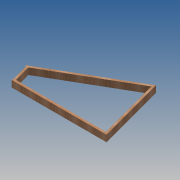
# Autodesk Inventor part: panelAflat
Saved by Autodesk Inventor 2014 SP1 (Build 180222100, 222)
## iProperties
Created: 2015-02-12
Part Number: panelAflat
Material: Wood (Birch)
Document SubType Name: Modeling
Designer: Dave
Density: 0.55 g/cm^3
Appearance: Birch - Natural Polished
Mass: 11299.2 g
Surface Area: 14418.2 cm^2
Volume: 20544 cm^3
Author: Dave
Autodesk Inventor part; units mm, degrees
ref_plane "YZ Plane" through (0, 0, 0) normal (1, 0, 0) x (0, 1, 0)
ref_plane "XZ Plane" through (0, 0, 0) normal (0, 1, 0) x (-1, 0, 0)
ref_plane "XY Plane" through (0, 0, 0) normal (0, 0, 1) x (1, 0, 0)
sketch "Sketch1" plane through (0, 0, 0) normal (0, 1, 0) x (-1, 0, 0)
  line L0 (0, 0) -> (-3000, 0) construction
  line L1 (0, 0) -> (-2598.0762, -1500) construction
  line L2 (0, 0) -> (3000, 0) construction
  arc A0 (-497.4937, 50) -> (-402.0602, -297.2332) centre (0, 0) ccw
  line L3 (-497.4937, 50) -> (-2157.4937, 50)
  line L4 (-2157.4937, 50) -> (-1841.7345, -1128.4295)
  line L5 (-2157.4937, 50) -> (-937.4937, 50) construction
  line L6 (-1841.7345, -1128.4295) -> (1158.2655, -1128.4295) construction
  line L7 (-1841.7345, -1128.4295) -> (-402.0602, -297.2332)
  arc A1 (-537.8662, 12) -> (-456.459, -284.7617) centre (0, 0) ccw
  line L8 (-2107.9712, 12) -> (-537.8662, 12)
  line L9 (-456.459, -284.7617) -> (-1817.8467, -1070.7593)
  line L10 (-2107.9712, 12) -> (-1817.8467, -1070.7593)
  dimension "d1" = 3000
  dimension "d2" = 150
  dimension "d3" = 1000
  dimension "d11" = 50
  dimension "d12" = 1660
  dimension "d13" = 1220
  dimension "d14" = 75
  constraints: 22 end point, 4 horizontal, 4 point on circle, 3 parallel, 2 centre point, 2 equal length, 1 coincident
  measures "d1" distance of L0.start L1.end
  measures "d2" angle of L1 L2
  measures "d3" diameter of A0
  measures "d11" distance between parallel lines of L3 L0
  measures "d12" distance of L3.start L3.end
  measures "d13" distance of L3.end L4.end
  measures "d14" angle of L4 L5
extrude "Extrusion2" add sketch "Sketch1" along normal blind 114
sketch "Sketch2" plane through (0, 114, 0) normal (0, 1, 0) x (1, 0, 0)
  line L0 (497.4937, -50) -> (2157.4937, -50) projected
  line L1 (1841.7345, 1128.4295) -> (402.0602, 297.2332) projected
  arc A0 (497.4937, -50) -> (402.0602, 297.2332) centre (0, 0) ccw projected
  line L2 (456.459, 284.7617) -> (537.8662, -12)
  line L3 (456.459, 284.7617) -> (423.5293, 265.7497)
  line L4 (537.8662, -12) -> (499.856, -12)
  line L5 (423.5293, 265.7497) -> (499.856, -12)
  constraints: 8 end point, 2 parallel, 2 point on circle
extrude "Extrusion3" add sketch "Sketch2" against normal blind 114 contours L5 A0
sketch "Sketch3" plane through (0, 114, 0) normal (0, 1, 0) x (1, 0, 0)
  arc A0 (537.8662, -12) -> (456.459, 284.7617) centre (0, 0) ccw projected
  line L0 (456.459, 284.7617) -> (537.8662, -12)
  constraints: 2 end point
extrude "Extrusion4" cut sketch "Sketch3" against normal blind 3500
sketch "Sketch4" plane through (0, 114, 0) normal (0, 1, 0) x (1, 0, 0)
  line L0 (537.8662, -12) -> (456.459, 284.7617) projected
  line L1 (2107.9712, -12) -> (537.8662, -12) projected
  line L2 (1841.7345, 1128.4295) -> (402.0602, 297.2332) projected
  line L3 (423.5293, 265.7497) -> (499.856, -12) projected
  line L4 (456.459, 284.7617) -> (423.5293, 265.7497)
  line L5 (499.856, -12) -> (537.8662, -12)
  constraints: 4 end point, 1 collinear, 1 parallel
extrude "Extrusion5" cut sketch "Sketch4" against normal blind 1
sketch "Sketch5" plane through (0, 114, 0) normal (0, 1, 0) x (1, 0, 0)
  line L0 (1817.8467, 1070.7593) -> (2107.9712, -12) projected
  line L1 (497.4937, -50) -> (2157.4937, -50) projected
  line L2 (2157.4937, -50) -> (1841.7345, 1128.4295) projected
  line L3 (1841.7345, 1128.4295) -> (402.0602, 297.2332) projected
  line L4 (1817.8467, 1070.7593) -> (1851.9166, 1090.4295)
  line L5 (2107.9712, -12) -> (2147.3116, -12)
  constraints: 4 end point, 2 parallel, 2 point on line
extrude "Extrusion6" cut sketch "Sketch5" against normal blind 1
body "Solid2"
